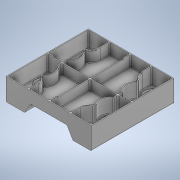
# Autodesk Inventor part: WarSunTray
Saved by Autodesk Inventor 2021 (Build 250183000, 183)
## iProperties
Created: 2023-03-17
Part Number: WarSunTray
Material: ABS Plastic
Document SubType Name: Modeling
Designer: Bradley
Density: 1.06 g/cm^3
Appearance: Smooth - Medium Gray
Author: Bradley
Autodesk Inventor part; units mm, degrees
ref_plane "YZ Plane" through (0, 0, 0) normal (1, 0, 0) x (0, 1, 0)
ref_plane "XZ Plane" through (0, 0, 0) normal (0, 1, 0) x (-1, 0, 0)
ref_plane "XY Plane" through (0, 0, 0) normal (0, 0, 1) x (1, 0, 0)
sketch "Sketch1" plane through (0, 0, 0) normal (0, 0, 1) x (1, 0, 0)
  line L0 (-74, 20.1) -> (-74, -17.9)
  line L1 (-74, -17.9) -> (-41.627, -17.9)
  line L2 (-41.627, -17.9) -> (-31.2924, 0)
  line L3 (-31.2924, 0) -> (31.2924, 0)
  line L4 (31.2924, 0) -> (41.627, -17.9)
  line L5 (41.627, -17.9) -> (74, -17.9)
  line L6 (74, -17.9) -> (74, 20.1)
  line L7 (-74, 20.1) -> (74, 20.1)
  line L8 (-31.2924, -0.5) -> (31.2924, -0.5) construction
  line L9 (31.2924, -0.5) -> (62.5848, -54.7) construction
  line L10 (62.5848, -54.7) -> (31.2924, -108.9) construction
  line L11 (31.2924, -108.9) -> (-31.2924, -108.9) construction
  line L12 (-31.2924, -108.9) -> (-62.5848, -54.7) construction
  line L13 (-62.5848, -54.7) -> (-31.2924, -0.5) construction
  line L14 (-74, -13.9) -> (-40.4723, -13.9)
  line L15 (-40.4723, -13.9) -> (-20.8423, 20.1)
  point P0 (0, 0)
  point P1 (0, 0)
  point P2 (0, 20.1)
  point P3 (0, -54.7)
  dimension "d0" = 74
  dimension "d2" = 38
  dimension "d3" = 108.4
  dimension "d4" = 0.5
  dimension "d5" = 0.25
  dimension "d6" = 91
  dimension "d53" = 20.1
  dimension "d115" = 4
  dimension "d116" = 1
  constraints: 32 end point, 4 point on line, 3 parallel, 3 perpendicular, 2 horizontal, 2 midpoint, 2 vertical alignment, 1 coincident, 1 collinear, 1 vertical, 13 other
  measures "d0" distance from line of point (0, 0) L0
  measures "d2" distance of L0.start L0.end
  measures "d3" distance between parallel lines of L11 L8
  measures "d4" distance between parallel lines of L8 L3
  measures "d5" distance between parallel lines of L13 L2
  measures "d6" distance between parallel lines of L11 L1
  measures "d53" distance between parallel lines of L3 L7
  measures "d115" distance between parallel lines of L1 L14
  measures "d116" distance between parallel lines of L2 L15
extrude "Extrusion1" add sketch "Sketch1" along normal mid plane 142.25
fillet "Fillet1" radius 2 6 edges at (-31.2924, 0, 0) (31.2924, 0, 0) (41.627, -17.9, 0) (-41.627, -17.9, 0) (-74, -17.9, 0) (74, -17.9, 0)
sketch "Sketch2" plane through (-74, 20.1, 71.125) normal (0, 1, 0) x (1, 0, 0)
  line L0 (0, 142.25) -> (0, 0) projected
  line L1 (148, 0) -> (0, 0) projected
  line L2 (148, 142.25) -> (148, 0) projected
  line L3 (0, 142.25) -> (148, 142.25) projected
  circle A0 centre (20.5, 125.35) radius 16 construction
  circle A1 centre (20.5, 125.35) radius 16.5 construction
  circle A2 centre (20.5, 125.35) radius 11.5 construction
  circle A3 centre (20.5, 125.35) radius 11.75
  circle A4 centre (20.5, 125.35) radius 16.9 construction
  line L4 (0, 142.25) -> (148, 142.25) construction
  line L5 (148, 142.25) -> (148, 0) construction
  line L6 (148, 0) -> (0, 0) construction
  line L7 (0, 142.25) -> (0, 0) construction
  line L8 (20.5, 125.35) -> (20.5, 141.85) construction
  line L9 (3.6, 140.65) -> (35, 140.65)
  line L10 (37, 138.65) -> (37, 125.35)
  line L11 (25, 71.925) -> (3.6, 71.925)
  line L12 (1.6, 73.925) -> (1.6, 138.65)
  arc A5 (3.6, 140.65) -> (1.6, 138.65) centre (3.6, 138.65) ccw
  arc A6 (37, 138.65) -> (35, 140.65) centre (35, 138.65) ccw
  arc A7 (1.6, 73.925) -> (3.6, 71.925) centre (3.6, 73.925) ccw
  line L13 (32.9504, 142.25) -> (32.9504, 0) projected
  line L14 (31.2183, 0) -> (31.2183, 142.25) projected
  circle A8 centre (16.9, 93.5531) radius 16.9 construction
  circle A9 centre (16.9, 93.5531) radius 16.5 construction
  circle A10 centre (16.9, 93.5531) radius 16 construction
  circle A11 centre (16.9, 93.5531) radius 11.75
  line L15 (26.543, 37.2404) -> (20.9266, 95.2817) construction
  line L16 (20.9266, 95.2817) -> (68.3836, 129.1663) construction
  line L17 (68.3836, 129.1663) -> (121.457, 105.0096) construction
  line L18 (121.457, 105.0096) -> (127.0734, 46.9683) construction
  line L19 (127.0734, 46.9683) -> (79.6164, 13.0837) construction
  line L20 (79.6164, 13.0837) -> (26.543, 37.2404) construction
  arc A12 (8.9852, 93.4488) -> (26.0637, 42.1938) centre (106.1816, 97.3624) ccw construction
  arc A13 (8.9852, 93.4488) -> (21.6672, 87.6277) centre (25.1434, 111.9261) ccw construction
  circle A14 centre (20.5, 125.35) radius 4 construction
  circle A15 centre (16.9, 93.5531) radius 4 construction
  circle A16 centre (16.9, 48.6969) radius 4 construction
  line L21 (16.9, 93.5531) -> (16.9, 48.6969) construction
  circle A17 centre (16.9, 93.5531) radius 4.4083 construction
  circle A18 centre (16.9, 48.6969) radius 4.4083 construction
  arc A19 (26.6774, 140.65) -> (14.3226, 140.65) centre (20.5, 125.35) ccw
  arc A20 (1.6, 99.7305) -> (1.6, 87.3758) centre (16.9, 93.5531) ccw
  line L22 (74, 71.125) -> (26.0731, 36.905)
  line L23 (26.0731, 36.905) -> (20.4011, 95.5209)
  line L24 (20.4011, 95.5209) -> (74, 71.125)
  arc A21 (8.4448, 94.6241) -> (25.5784, 42.017) centre (106.1816, 97.3624) ccw
  arc A22 (8.4448, 94.6241) -> (21.1075, 88.2214) centre (25.1434, 111.9261) ccw
  line L25 (25, 71.925) -> (25, 79.1782)
  arc A23 (25, 79.1782) -> (27.3987, 106.2822) centre (16.9, 93.5531) ccw
  arc A24 (27.8871, 110.596) -> (37, 125.35) centre (20.5, 125.35) ccw
  line L26 (20.5, 125.35) -> (16.9, 93.5531) construction
  line L27 (27.8871, 110.596) -> (27.3987, 106.2822)
  point P0 (16.9, 71.125)
  dimension "d10" = 32
  dimension "d13" = 23
  dimension "d23" = 0.4
  dimension "d26" = 23.5
  dimension "d27" = 33
  dimension "d28" = 2
  dimension "d70" = 4.9765
  dimension "d71" = 7.6898
  dimension "d72" = 101
  dimension "d73" = 97.2752
  dimension "d74" = 24.5458
  dimension "d75" = 8
  dimension "d76" = 12.0624
  dimension "d77" = 5.4473
  dimension "d78" = 1.6
  dimension "d79" = 1.6
  dimension "d80" = 0.8
  dimension "d81" = 20.5
  dimension "d84" = 0.5
  dimension "d85" = 0.5
  dimension "d86" = 0.5
  dimension "d106" = 25
  dimension "d107" = 9
  constraints: 36 end point, 31 point on circle, 25 centre point, 12 coincident, 12 tangent, 11 equal radius, 10 point on line, 4 concentric, 4 parallel, 3 vertical, 1 horizontal, 1 horizontal alignment, 1 midpoint, 1 perpendicular, 1 vertical alignment, 13 other
  measures "d10" diameter of A0
  measures "d13" diameter of A2
  measures "d23" radial gap between concentric circles of A1 A4
  measures "d26" diameter of A3
  measures "d27" diameter of A1
  measures "d28" radius of A5
  measures "d70" distance of L15.start A12.end
  measures "d71" distance of A13.end L15.end
  measures "d72" distance between parallel lines of L18 L15
  measures "d73" radius of A12
  measures "d74" radius of A13
  measures "d75" diameter of A14
  measures "d76" distance from line of A12.start L15
  measures "d77" distance from line of A12.start L16
  measures "d78" distance between parallel lines of L9 L3
  measures "d79" distance between parallel lines of L12 L0
  measures "d80" distance from line of L11 point (16.9, 71.125)
  measures "d81" distance from line of A0.centre L0
  measures "d84" distance between parallel lines of L15 L23
  measures "d85" radial gap between concentric circles of A12 A21
  measures "d86" radial gap between concentric circles of A13 A22
  measures "d106" distance between parallel lines of L0 L25
  measures "d107" distance between parallel lines of L27 L26
extrude "Extrusion2" cut sketch "Sketch2" against normal blind 37 contours L14 A3 | A3 L14 | L24 L23 A22 A21 A11 | A11 L23 L24 | A11 A21 A22 L23
extrude "Extrusion3" cut sketch "Sketch2" against normal blind 27 contours L14 A3 A24 L27 A23 L24 A11 A21 L11 A7 L12 A5 L9 | L9 L13 A24 L14 A3 | L9 A6 L10 A24 L13 | L14 A3 | A3 L14 | A23 L25 L11 L23 A11 L24 L14 | L14 L24 L13 A23 | L13 L24 A23 | L14 A23 L13 L24 | A23 L24 L13 | L24 L23 A22 A21 A11 | A11 L23 L24 | L11 A21 A11 L23 | A11 A21 A22 L23
chamfer "Chamfer1" distance 2 angle 45 2 edges at (-65.25, -6.9, -54.225) (-68.85, -6.9, -22.4281)
fillet "Fillet3" radius 1 17 edges at (-65.25, -16.9, -54.225) (-65.25, -8.9, -54.225) (-67.25, -6.9, -54.225) (-39.4619, -6.9, -45.5543) (-71.8142, -6.9, -68.9392) (-72.4, -6.9, -35.1625) (-54.7, -6.9, -69.525) (-37.5858, -6.9, -68.9392) (-37, -6.9, -60.875) (-59.7, -6.9, -0.8) (-71.8142, -6.9, -1.3858) (-40.6642, -6.9, -20.9736) (-70.85, -6.9, -22.4281) (-68.85, -8.9, -22.4281) (-68.85, -16.9, -22.4281) (-46.3571, -6.9, -37.3141) (-49, -6.9, -4.4266)
fillet "Fillet3" radius 2 1 edges at (-49, 6.6, -0.8)
fillet "Fillet3" radius 3 3 edges at (-46.6013, 6.6, -35.1572) (-46.1129, 6.6, -39.471) (-49, 6.6, -8.0532)
sketch "Sketch6" plane through (-74, 20.1, 71.125) normal (0, 1, 0) x (1, 0, 0)
  arc A0 (26.2923, 79.9872) -> (25, 77.5207) centre (28, 77.5207) ccw projected
  line L0 (25, 77.5207) -> (25, 73.925) projected
  arc A1 (23, 71.925) -> (25, 73.925) centre (23, 73.925) ccw projected
  line L1 (23, 71.925) -> (3.6, 71.925) projected
  arc A2 (1.6, 73.925) -> (3.6, 71.925) centre (3.6, 73.925) ccw projected
  line L2 (1.6, 73.925) -> (1.6, 138.65) projected
  arc A3 (3.6, 140.65) -> (1.6, 138.65) centre (3.6, 138.65) ccw projected
  line L3 (3.6, 140.65) -> (35, 140.65) projected
  arc A4 (37, 138.65) -> (35, 140.65) centre (35, 138.65) ccw projected
  line L4 (37, 138.65) -> (37, 125.35) projected
  arc A5 (29.1262, 111.2845) -> (37, 125.35) centre (20.5, 125.35) ccw projected
  arc A6 (29.1262, 111.2845) -> (27.7137, 109.0646) centre (30.6946, 108.7271) ccw projected
  line L5 (27.7137, 109.0646) -> (27.572, 107.8135) projected
  arc A7 (27.572, 107.8135) -> (28.4525, 105.334) centre (30.553, 107.476) ccw projected
  arc A8 (26.2923, 79.9872) -> (28.4525, 105.334) centre (16.9, 93.5531) ccw projected
  line L6 (0, 142.25) -> (0, 0) projected
  line L7 (148, 0) -> (0, 0) projected
  line L8 (148, 142.25) -> (148, 0) projected
  line L9 (0, 142.25) -> (148, 142.25) projected
  line L10 (38.6, 125.35) -> (38.6, 138.65)
  arc A9 (38.6, 138.65) -> (33.6952, 142.0052) centre (35, 138.65) ccw
  line L11 (33.6952, 142.0052) -> (27.6776, 142.0052)
  arc A10 (27.8624, 142.4398) -> (27.6776, 142.0052) centre (30.8912, 140.8951) ccw
  arc A11 (27.8624, 142.4398) -> (15.9376, 142.4398) centre (21.9, 125.35) ccw
  arc A12 (14.8176, 142.25) -> (15.9376, 142.4398) centre (14.8176, 145.65) ccw
  line L12 (14.8176, 142.25) -> (3.6, 142.25)
  arc A13 (3.6, 142.25) -> (0, 138.65) centre (3.6, 138.65) ccw
  line L13 (0, 138.65) -> (0, 100.3193)
  arc A14 (-0.1898, 99.1993) -> (0, 100.3193) centre (-3.4, 100.3193) ccw
  arc A15 (-0.1898, 99.1993) -> (-0.1898, 87.2745) centre (16.9, 93.2369) ccw
  arc A16 (0, 86.1545) -> (-0.1898, 87.2745) centre (-3.4, 86.1545) ccw
  line L14 (0, 86.1545) -> (0, 73.925)
  arc A17 (0, 73.925) -> (3.6, 70.325) centre (3.6, 73.925) ccw
  line L15 (3.6, 70.325) -> (23, 70.325)
  arc A18 (23, 70.325) -> (26.6, 73.925) centre (23, 73.925) ccw
  line L16 (26.6, 73.925) -> (26.6, 77.5207)
  arc A19 (27.2031, 78.6717) -> (26.6, 77.5207) centre (28, 77.5207) ccw
  arc A20 (27.2031, 78.6717) -> (29.5728, 106.4764) centre (16.9, 93.5531) ccw
  arc A21 (29.1619, 107.6335) -> (29.5728, 106.4764) centre (30.553, 107.476) ccw
  line L17 (29.1619, 107.6335) -> (29.3035, 108.8846)
  arc A22 (29.9627, 109.9206) -> (29.3035, 108.8846) centre (30.6946, 108.7271) ccw
  arc A23 (29.9627, 109.9206) -> (38.6, 125.35) centre (20.5, 125.35) ccw
  arc A24 (40.6, 140.65) -> (38.6, 138.65) centre (40.6, 138.65) ccw
  arc A25 (26.6, 73.925) -> (28.6, 71.925) centre (28.6, 73.925) ccw
  arc A26 (71.2, 71.925) -> (73.2, 73.925) centre (71.2, 73.925) ccw
  arc A27 (73.2, 138.65) -> (71.2, 140.65) centre (71.2, 138.65) ccw
  line L18 (40.6, 140.65) -> (71.2, 140.65)
  line L19 (73.2, 138.65) -> (73.2, 73.925)
  line L20 (71.2, 71.925) -> (28.6, 71.925)
  line L21 (43.8623, 142.25) -> (43.8623, 0) projected
  line L22 (38.3326, 122.25) -> (43.8623, 122.25)
  point P0 (74, 71.125)
  point P1 (43.8623, 71.925)
  point P2 (43.8623, 140.65)
  dimension "d110" = 0.8
  dimension "d121" = 20
  constraints: 39 point on circle, 24 end point, 19 centre point, 8 tangent, 2 collinear, 2 equal radius, 1 parallel, 1 perpendicular, 1 point on line, 1 vertical, 12 other
  measures "d110" distance from line of point (74, 71.125) L19
  measures "d121" distance between parallel lines of L22 L9
extrude "Extrusion8" cut sketch "Sketch6" against normal blind 19.1 contours A24 L18 L21 L22 A23 L10 | L18 A27 L19 A26 L20 L21 | L20 A25 L16 A19 A20 A21 L17 A22 A23 L22 L21
fillet "Fillet4" radius 1 8 edges at (-1.3858, 1, -1.3858) (-0.8, 1, -35.1625) (-1.3858, 1, -68.9392) (-18.1, 1, -69.525) (-34.8142, 1, -68.9392) (-35.4, 1, -60.875) (-37.7062, 1, -45.3838) (-24.1, 1, -0.8)
mirror "Mirror1" about plane through (0, 0, 0) normal (1, 0, 0) of "Extrusion2", "Extrusion3", "Chamfer1", "Fillet3", "Extrusion8", "Fillet4"
mirror "Mirror2" about plane through (0, 0, 0) normal (0, 0, 1) of "Extrusion2", "Extrusion3", "Chamfer1", "Fillet3", "Mirror1", "Extrusion8", "Fillet4"
extrude "Extrusion6" cut sketch "Sketch2" against normal blind 2 contours L22 L23 L11 L25 A23 L14 | L14 A23 L13 L22 | L13 A23 L24 L22 | A23 L25 L11 L23 A11 L24 L14 | L14 L24 L13 A23 | L13 L24 A23 | A21 L11 L23 | A11 L23 L24 | L11 A21 A11 L23 | A11 A21 A22 L23 picked at (31.4569, 87.5684) picked at (32.9523, 89.7631)
pattern_circular "Circular Pattern1" count 6 over 360 about axis through (0, -10, 0) along (0, 1, 0) of "Extrusion6"
equation "\"d2\" = Depth"
equation "\"d3\" = Outside"
equation "\"Depth\" = 38"
equation "\"Outside\" = 108.4"
body "Solid1"
